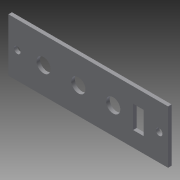
# Autodesk Inventor part: switch and led mount cap
Saved by Autodesk Inventor 2014 SP1 (Build 180222100, 222)
## iProperties
Created: 2017-06-27
Part Number: switch and led mount cap
Material: Generic
Document SubType Name: Modeling
Designer: kteo17
Density: 1 g/cm^3
Appearance: Default
Author: kteo17
Autodesk Inventor part; units mm, degrees
ref_plane "YZ Plane" through (0, 0, 0) normal (1, 0, 0) x (0, 1, 0)
ref_plane "XZ Plane" through (0, 0, 0) normal (0, 1, 0) x (-1, 0, 0)
ref_plane "XY Plane" through (0, 0, 0) normal (0, 0, 1) x (1, 0, 0)
sketch "Sketch1" plane through (0, 0, 0) normal (0, 0, 1) x (1, 0, 0)
  circle A0 centre (25.0551, 9.5259) radius 2.54
  line L0 (49.3502, 4.5729) -> (43.7622, 4.5729)
  line L1 (43.7622, 4.5729) -> (43.7622, 14.4789)
  line L2 (43.7622, 14.4789) -> (49.3502, 14.4789)
  line L3 (49.3502, 14.4789) -> (49.3502, 4.5729)
  circle A1 centre (37.5265, 9.5259) radius 2.54
  circle A2 centre (12.5837, 9.5259) radius 2.54
  circle A3 centre (53.973, 9.51) radius 1.1906
  circle A4 centre (3.173, 9.5259) radius 1.1906
  line L4 (-0.002, 19.0191) -> (57.148, 19.0191)
  line L5 (-0.002, 0.0009) -> (-0.002, 19.0191)
  line L6 (57.148, 0.0009) -> (-0.002, 0.0009)
  line L7 (57.148, 19.0191) -> (57.148, 0.0009)
  point P0 (0, 0)
  point P1 (6.348, 3.1759)
  dimension "d2" = 5.08
  dimension "d3" = 57.15
  dimension "d4" = 19.0182
  dimension "d5" = 3.175
  dimension "d6" = 3.175
  dimension "d7" = 5.588
  dimension "d8" = 9.906
  dimension "d9" = 4.572
  dimension "d10" = 7.7978
  dimension "d11" = 12.4714
  dimension "d12" = 12.4714
  dimension "d13" = 5.08
  dimension "d14" = 5.08
  constraints: 16 end point, 5 centre point
  measures "d2" diameter of A2
  measures "d3" distance of L4.start L4.end
  measures "d4" distance of L5.start L4.start
  measures "d5" distance from line of L5 A4.centre
  measures "d6" distance from line of L7 A3.centre
  measures "d7" distance between parallel lines of L1 L3
  measures "d8" distance between parallel lines of L0 L2
  measures "d9" distance between parallel lines of L6 L0
  measures "d10" distance between parallel lines of L7 L3
  measures "d11" distance of A0.centre A2.centre
  measures "d12" distance of A1.centre A0.centre
  measures "d13" diameter of A0
  measures "d14" diameter of A1
extrude "Extrusion1" add sketch "Sketch1" along normal blind 1.27
sketch "Sketch2" plane through (0, 0, 1.27) normal (0, 0, 1) x (1, 0, 0)
  line L0 (43.7622, 4.5729) -> (43.7622, 14.4789) projected
  line L1 (43.7622, 14.4789) -> (49.3502, 14.4789) projected
  line L2 (49.3502, 14.4789) -> (49.3502, 4.5729) projected
  line L3 (49.3502, 4.5729) -> (43.7622, 4.5729) projected
  line L4 (48.4612, 13.5899) -> (44.6512, 13.5899)
  line L5 (44.6512, 13.5899) -> (44.6512, 5.4619)
  line L6 (44.6512, 5.4619) -> (48.4612, 5.4619)
  line L7 (48.4612, 5.4619) -> (48.4612, 13.5899)
  point P0 (0, 0)
  dimension "d16" = 3.81
  constraints: 8 end point, 3 other
  measures "d16" distance of L4.start L4.end
extrude "Extrusion2" add sketch "Sketch2" against normal blind 2.54
sketch "Sketch3" plane through (0, 0, -1.27) normal (0, 0, -1) x (-1, 0, 0)
  line L0 (-44.6512, 13.5899) -> (-44.6512, 5.4619) projected
  line L1 (-44.6512, 5.4619) -> (-48.4612, 5.4619) projected
  line L2 (-48.4612, 5.4619) -> (-48.4612, 13.5899) projected
  line L3 (-48.4612, 13.5899) -> (-44.6512, 13.5899) projected
  line L4 (-43.7622, 4.5729) -> (-43.7622, 14.4789) projected
  line L5 (-43.7622, 14.4789) -> (-49.3502, 14.4789) projected
  line L6 (-49.3502, 14.4789) -> (-49.3502, 4.5729) projected
  line L7 (-49.3502, 4.5729) -> (-43.7622, 4.5729) projected
  point P0 (0, 0)
extrude "Extrusion3" cut sketch "Sketch3" against normal blind 1.27
body "Solid1"
